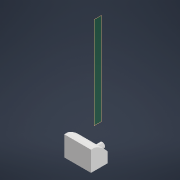
# Autodesk Inventor part: servo shaft
Saved by Autodesk Inventor 2021 (Build 250183000, 183)
## iProperties
Created: 2021-11-22
Part Number: servo shaft
Material: Generic
Document SubType Name: Modeling
Designer: techv
Density: 1 g/cm^3
Appearance: Default
Author: techv
Autodesk Inventor part; units mm, degrees
ref_plane "YZ Plane" through (0, 0, 0) normal (1, 0, 0) x (0, 1, 0)
ref_plane "XZ Plane" through (0, 0, 0) normal (0, 1, 0) x (-1, 0, 0)
ref_plane "XY Plane" through (0, 0, 0) normal (0, 0, 1) x (1, 0, 0)
ref_plane "Work Plane1" through (-65, -62.5, 0) normal (-1, 0, 0) x (0, 1, 0)
ref_plane "Work Plane2" through (-59, 26.5316, -72.121) normal (-1, 0, 0) x (0, -0.8294, 0.5586)
sketch "Sketch3" plane through (-59, 26.5316, -72.121) normal (-1, 0, 0) x (0, -0.8294, 0.5586)
  circle A0 centre (153.729, 98.9235) radius 2.5 projected
  line L0 (143.729, 118.9235) -> (159.8751, 108.0498) projected
  line L1 (143.729, 118.9235) -> (141.729, 118.9235) projected
  line L2 (141.729, 118.9235) -> (141.729, 78.9235) projected
  line L3 (143.729, 78.9235) -> (141.729, 78.9235) projected
  line L4 (159.8751, 89.7972) -> (143.729, 78.9235) projected
  arc A1 (159.8751, 89.7972) -> (159.8751, 108.0498) centre (153.729, 98.9235) ccw projected
  circle A2 centre (153.729, 98.9235) radius 2.5 projected
  line L5 (165.729, 118.9235) -> (141.729, 118.9235)
  line L6 (141.729, 118.9235) -> (141.729, 78.9235)
  line L7 (141.729, 78.9235) -> (165.729, 78.9235)
  line L8 (165.729, 78.9235) -> (165.729, 118.9235)
  line L9 (165.729, 118.9235) -> (141.729, 78.9235) construction
  line L10 (141.729, 118.9235) -> (165.729, 78.9235) construction
  point P0 (62.2926, 45)
  constraints: 12 end point, 2 midpoint, 2 parallel, 1 horizontal, 1 perpendicular
extrude "Extrusion3" add sketch "Sketch3" along normal blind 12 contours A0 | L5 L8 L7 L4 A1 L0 | L0 A1 L4 L3 L2 L1
body "Solid2"
